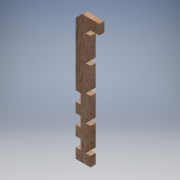
# Autodesk Inventor part: MarkerShaft
Saved by Autodesk Inventor 2019 (Build 230136000, 136)
## iProperties
Created: 2019-01-14
Part Number: MarkerShaft
Material: Wood (Birch)
Document SubType Name: Modeling
Designer: nxgam
Density: 0.55 g/cm^3
Appearance: Birch - Natural Polished
Author: nxgam
Autodesk Inventor part; units mm, degrees
ref_plane "YZ Plane" through (0, 0, 0) normal (1, 0, 0) x (0, 1, 0)
ref_plane "XZ Plane" through (0, 0, 0) normal (0, 1, 0) x (-1, 0, 0)
ref_plane "XY Plane" through (0, 0, 0) normal (0, 0, 1) x (1, 0, 0)
sketch "Sketch1" plane through (0, 0, 0) normal (0, 0, 1) x (1, 0, 0)
  line L0 (0, 0) -> (10.16, 0)
  line L1 (10.16, 0) -> (10.16, 132.08)
  line L2 (10.16, 132.08) -> (0, 132.08)
  line L3 (0, 132.08) -> (0, 0)
  line L4 (10.16, 10.16) -> (5.08, 10.16)
  line L5 (5.08, 10.16) -> (5.08, 15.24)
  line L6 (5.08, 15.24) -> (10.16, 15.24)
  line L7 (10.16, 15.24) -> (10.16, 10.16)
  line L8 (10.16, 36.83) -> (5.08, 36.83)
  line L9 (5.08, 36.83) -> (5.08, 41.91)
  line L10 (5.08, 41.91) -> (10.16, 41.91)
  line L11 (10.16, 41.91) -> (10.16, 36.83)
  line L12 (10.16, 63.5) -> (5.08, 63.5)
  line L13 (5.08, 63.5) -> (5.08, 68.58)
  line L14 (5.08, 68.58) -> (10.16, 68.58)
  line L15 (10.16, 68.58) -> (10.16, 63.5)
  line L16 (10.16, 90.17) -> (5.08, 90.17)
  line L17 (5.08, 90.17) -> (5.08, 95.25)
  line L18 (5.08, 95.25) -> (10.16, 95.25)
  line L19 (10.16, 95.25) -> (10.16, 90.17)
  line L20 (10.16, 116.84) -> (5.08, 116.84)
  line L21 (5.08, 116.84) -> (5.08, 121.92)
  line L22 (5.08, 121.92) -> (10.16, 121.92)
  line L23 (10.16, 121.92) -> (10.16, 116.84)
  dimension "d0" = 10.16
  dimension "d1" = 132.08
  dimension "d2" = 5.08
  dimension "d3" = 5.08
  dimension "d4" = 10.16
  dimension "d7" = 26.67
  constraints: 48 end point, 4 parallel, 2 horizontal, 2 perpendicular, 1 point on line, 1 vertical, 32 other
  measures "d0" distance of L2.end L1.end
  measures "d1" distance of L1.end L0.end
  measures "d2" distance of L5.end L6.end
  measures "d3" distance of L4.end L5.end
  measures "d4" distance between parallel lines of L0 L4
  measures "d7" distance of L4.start L8.start
extrude "Extrusion2" add sketch "Sketch1" along normal blind 5.08 contours L3 L2 L1 L22 L21 L20 L18 L17 L16 L14 L13 L12 L10 L9 L8 L6 L5 L4 L0
thicken "Thicken3" operation add thickness 5.08 both sides no extend neighbours yes toward (-1, 0, 0) faces at (0, 88.0533, 1.6933)
thicken "Thicken4" operation add thickness 8.89 both sides no extend neighbours yes toward (1, 0, 0) faces at (10.16, 125.3067, 3.3867)
chamfer "Chamfer2" distance 6.35 angle 45 1 edges at (-5.08, 132.08, 2.54)
sketch "Sketch2" plane through (0, 0, 5.08) normal (0, 0, 1) x (1, 0, 0)
  line L0 (-5.08, -3.4261) -> (-5.08, 0)
  line L1 (-5.08, 0) -> (0, 0)
  line L2 (0, 0) -> (0, -3.4261)
  line L3 (0, -3.4261) -> (-5.08, -3.4261)
  line L4 (-5.08, 10.16) -> (-5.08, 20.32)
  line L5 (-5.08, 20.32) -> (0, 20.32)
  line L6 (0, 20.32) -> (0, 10.16)
  line L7 (0, 10.16) -> (-5.08, 10.16)
  line L8 (-5.08, 30.48) -> (-5.08, 40.64)
  line L9 (-5.08, 40.64) -> (0, 40.64)
  line L10 (0, 40.64) -> (0, 30.48)
  line L11 (0, 30.48) -> (-5.08, 30.48)
  line L12 (-5.08, 50.8) -> (-5.08, 60.96)
  line L13 (-5.08, 60.96) -> (0, 60.96)
  line L14 (0, 60.96) -> (0, 50.8)
  line L15 (0, 50.8) -> (-5.08, 50.8)
  constraints: 32 end point, 8 horizontal, 8 vertical, 15 other
extrude "Extrusion3" cut sketch "Sketch2" against normal blind 5.08 contours L4 L5 L6 L7 | L8 L9 L10 L11 | L12 L13 L14 L15
body "Solid2"
